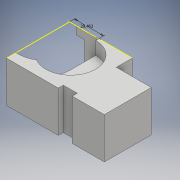
# Autodesk Inventor part: Part1
Saved by Autodesk Inventor 2017 (Build 210142000, 142)
## iProperties
Created: 2019-09-25
Part Number: Part1
Material: Generic
Document SubType Name: Modeling
Designer: STUDENT04
Density: 1 g/cm^3
Appearance: Default
Author: STUDENT04
Autodesk Inventor part; units mm, degrees
ref_plane "YZ Plane" through (0, 0, 0) normal (1, 0, 0) x (0, 1, 0)
ref_plane "XZ Plane" through (0, 0, 0) normal (0, 1, 0) x (-1, 0, 0)
ref_plane "XY Plane" through (0, 0, 0) normal (0, 0, 1) x (1, 0, 0)
sketch "Sketch1" plane through (0, 0, 0) normal (0, 0, 1) x (1, 0, 0)
  line L0 (-15.8942, -5.4427) -> (36.1058, -5.4427)
  line L1 (36.1058, -5.4427) -> (36.1058, -0.4427)
  line L2 (36.1058, -0.4427) -> (50.1058, -0.4427)
  line L3 (50.1058, -0.4427) -> (50.1058, -5.4427)
  line L4 (50.1058, -5.4427) -> (82.1058, -5.4427)
  line L5 (82.1058, -5.4427) -> (82.1058, 41.5573)
  line L6 (82.1058, 41.5573) -> (47.1058, 41.5573)
  line L7 (47.1058, 41.5573) -> (47.1058, 57.5573)
  line L8 (47.1058, 57.5573) -> (13.1058, 57.5573)
  line L9 (13.1058, 57.5573) -> (-15.8942, 57.5573)
  line L10 (-15.8942, 57.5573) -> (-15.8942, -5.4427)
  point P0 (0, 0)
  dimension "d0" = 52
  dimension "d1" = 5
  dimension "d2" = 14
  dimension "d3" = 5
  dimension "d4" = 32
  dimension "d5" = 47
  dimension "d6" = 35
  dimension "d7" = 16
  dimension "d8" = 34
  dimension "d9" = 29
  constraints: 22 end point, 5 perpendicular, 3 point on line, 1 horizontal, 1 vertical
  measures "d0" distance of L0.start L0.end
  measures "d1" distance of L0.end L1.end
  measures "d2" distance of L1.end L2.end
  measures "d3" distance of L2.end L3.end
  measures "d4" distance of L3.end L4.end
  measures "d5" distance of L4.end L5.end
  measures "d6" distance of L5.end L6.end
  measures "d7" distance of L6.end L7.end
  measures "d8" distance of L7.end L8.end
  measures "d9" distance of L8.end L9.end
extrude "Extrusion1" add sketch "Sketch1" along normal blind 41
sketch "Sketch10" plane through (0, 0, 41) normal (0, 0, 1) x (1, 0, 0)
  line L0 (-15.8942, 57.5573) -> (-15.8942, -5.4427) projected
  line L1 (47.1058, 57.5573) -> (-15.8942, 57.5573) projected
  point P0 (0, 0)
  point P1 (13.569, 57.5573)
  dimension "d16" = 29.4632
  constraints: 1 point on line
  measures "d16" distance of L0.start point (13.569, 57.557)
sketch "Sketch12" plane through (0, 0, 41) normal (0, 0, 1) x (1, 0, 0)
  circle A0 centre (-80.4891, 35.6187) radius 25
  line L0 (47.1058, 57.5573) -> (-15.8942, 57.5573) projected
  circle A1 centre (13.4877, 29.5573) radius 25
  point P0 (0, 0)
  dimension "d17" = 50
  dimension "d18" = 50
  dimension "d19" = 28
  constraints: 2 centre point
  measures "d17" diameter of A0
  measures "d18" diameter of A1
  measures "d19" distance from line of L0 A1.centre
extrude "Extrusion2" cut sketch "Sketch12" against normal blind 13 contours A1
sketch "Sketch13" plane through (0, 0, 41) normal (0, 0, 1) x (1, 0, 0)
  circle A0 centre (-18.8292, 31.3442) radius 32
  circle A1 centre (13.4877, 29.5573) radius 25 projected
  line L0 (13.4877, 54.5573) -> (13.4877, 4.5573)
  circle A2 centre (-13.4781, 30.9626) radius 27
  point P0 (0, 0)
  dimension "d22" = 64
  dimension "d23" = 54
  constraints: 2 centre point, 2 end point, 2 point on circle
  measures "d22" diameter of A0
  measures "d23" diameter of A2
extrude "Extrusion3" cut sketch "Sketch13" against normal through all contours A0 A2 A1 | A0 A2 L0 | A2 L0 | A1 A2 picked at (-3.1402, 31.014)
sketch "Sketch14" plane through (0, 0, 41) normal (0, 0, 1) x (1, 0, 0)
  arc A0 (0.7748, 8.031) -> (3.0811, 52.2884) centre (-13.4781, 30.9626) ccw projected
  line L0 (13.5219, 30.9626) -> (13.5219, 57.5526)
  line L1 (13.5219, 57.5526) -> (-18.1655, 57.5526)
  line L2 (-18.1655, 57.5526) -> (13.5219, 30.9626)
  point P0 (0, 0)
  dimension "d26" = 41.3657
  dimension "d27" = 31.6874
  constraints: 6 end point, 2 point on circle, 1 perpendicular, 1 point on line, 1 tangent, 1 vertical
  measures "d26" distance of L1.end L2.end
  measures "d27" distance of L0.end L1.end
extrude "Extrusion4" cut sketch "Sketch14" against normal through all
sketch "Sketch15" plane through (0, 0, 41) normal (0, 0, 1) x (1, 0, 0)
  point P0 (0, 0)
sketch "Sketch16" plane through (0, 0, 0) normal (0, 0, -1) x (-1, 0, 0)
  circle A0 centre (18.3913, 30.8453) radius 32
  point P0 (0, 0)
  dimension "d30" = 64
  constraints: 1 centre point
  measures "d30" diameter of A0
extrude "Extrusion5" cut sketch "Sketch16" against normal blind 33
sketch "Sketch21" plane through (47.1058, 57.5573, 41) normal (0, 1, 0) x (1, 0, 0)
  line L0 (0, 41) -> (-47.877, 41) projected
  line L1 (-63, 8) -> (-63, 41) projected
  point P0 (-47.1058, 41)
  point P1 (-25, 25)
  dimension "d33" = 16
  dimension "d34" = 38
  measures "d33" distance from line of point (-25, 25) L0
  measures "d34" distance from line of point (-25, 25) L1
hole "Hole1" at (22.1058, 57.5573, 16) direction (0, -1, 0) diameter 9.376 depth 29.3 tip angle 118 thread size "M11x1.5" class "6H" standard "ANSI Metric M Profile"
sketch "Sketch22" plane through (47.1058, 57.5573, 41) normal (0, 1, 0) x (1, 0, 0)
  point P0 (-47.1058, 41)
body "Solid1"
